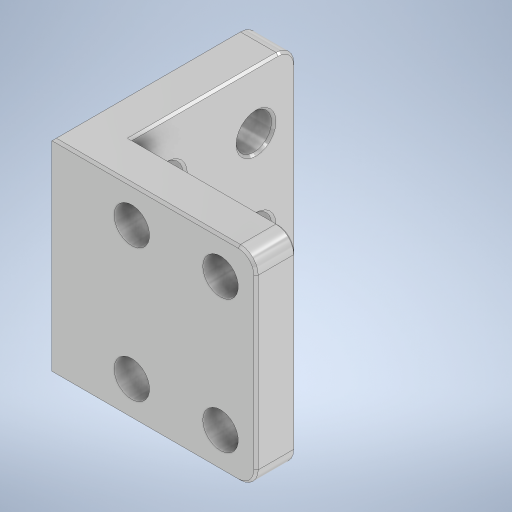
# Autodesk Inventor part: HUDSON-1-06 FRONT BUFFER BEAM ANGLE
Saved by Autodesk Inventor 2024.2 (Build 282272000, 272)
## iProperties
Created: 2024-10-05
Part Number: HUDSON-1-06 FRONT BUFFER BEAM ANGLE
Material: Generic
Document SubType Name: Modeling
Designer: Jimena Brenes
Density: 1 g/cm^3
Appearance: Aluminum - Dark
Author: Jimena Brenes
Autodesk Inventor part; units mm, degrees
ref_plane "YZ Plane" through (0, 0, 0) normal (1, 0, 0) x (0, 1, 0)
ref_plane "XZ Plane" through (0, 0, 0) normal (0, 1, 0) x (-1, 0, 0)
ref_plane "XY Plane" through (0, 0, 0) normal (0, 0, 1) x (1, 0, 0)
sketch "Sketch1" plane through (0, 0, 0) normal (0, 1, 0) x (-1, 0, 0)
  line L0 (0, 0) -> (0, -4.5)
  line L1 (0, 0) -> (23, 0)
  line L2 (23, 0) -> (23, -23)
  line L3 (23, -23) -> (18.5, -23)
  line L4 (0, -4.5) -> (18.5, -4.5)
  line L5 (18.5, -4.5) -> (18.5, -23)
  dimension "d0" = 4.5
  dimension "d1" = 23
  dimension "d2" = 23
  dimension "d3" = 4.5
  constraints: 12 end point, 3 perpendicular, 2 horizontal, 1 vertical
  measures "d0" distance of L0.start L0.end
  measures "d1" distance of L0.start L1.end
  measures "d2" distance of L1.end L2.end
  measures "d3" distance of L2.end L3.end
extrude "Extrusion1" add sketch "Sketch1" along normal blind 23
fillet "Fillet1" radius 2 4 edges at (-20.75, 23, -23) (-20.75, 0, -23) (0, 0, -2.25) (0, 23, -2.25)
sketch "Sketch2" plane through (-18.5, 0, -4.5) normal (0, 0, -1) x (-1, 0, 0)
  circle A0 centre (-14.5, 19) radius 2
  circle A1 centre (-4.5, 19) radius 2
  circle A2 centre (-4.5, 4) radius 2
  circle A3 centre (-14.5, 4) radius 2
  line L0 (-16.5, 23) -> (0, 23) projected
  line L1 (-16.5, 0) -> (0, 0) projected
  line L2 (-18.5, 2) -> (-18.5, 21) projected
  line L3 (4.5, 2) -> (4.5, 21) projected
  point P0 (-18.5, 0)
  dimension "d7" = 4
  dimension "d8" = 4
  dimension "d9" = 4
  dimension "d10" = 4
  dimension "d11" = 4
  dimension "d12" = 15
  dimension "d13" = 4
  dimension "d14" = 4
  dimension "d15" = 10
  dimension "d16" = 4
  dimension "d17" = 4
  dimension "d18" = 9
  dimension "d19" = 9
  constraints: 4 centre point
  measures "d7" diameter of A0
  measures "d8" diameter of A1
  measures "d9" diameter of A2
  measures "d10" diameter of A3
  measures "d11" distance from line of L0 A0.centre
  measures "d12" distance of A3.centre A0.centre
  measures "d13" distance from line of L1 A3.centre
  measures "d14" distance from line of L2 A3.centre
  measures "d15" distance of A3.centre A2.centre
  measures "d16" distance from line of L1 A2.centre
  measures "d17" distance from line of L0 A1.centre
  measures "d18" distance from line of L3 A1.centre
  measures "d19" distance from line of L3 A2.centre
hole "Hole1" at (-4, 19, -4.5) at (-4, 4, -4.5) at (-14, 19, -4.5) at (-14, 4, -4.5) direction (0, 0, 1) diameter 4 depth 4.5 tip angle 118
sketch "Sketch3" plane through (-18.5, 0, -4.5) normal (1, 0, 0) x (0, 0, -1)
  line L0 (4, 16.5) -> (14, 16.5) construction
  line L1 (14, 16.5) -> (14, 6.5) construction
  line L2 (14, 6.5) -> (4, 6.5) construction
  line L3 (4, 6.5) -> (4, 16.5) construction
  circle A0 centre (4, 16.5) radius 2
  circle A1 centre (14, 16.5) radius 2
  circle A2 centre (14, 6.5) radius 2
  circle A3 centre (4, 6.5) radius 2
  line L4 (0, 23) -> (16.5, 23) projected
  line L5 (-4.5, 2) -> (-4.5, 21) projected
  line L6 (18.5, 2) -> (18.5, 21) projected
  point P0 (-4.5, 0)
  dimension "d27" = 4
  dimension "d28" = 4
  dimension "d29" = 4
  dimension "d30" = 4
  dimension "d31" = 6.5
  dimension "d32" = 10
  dimension "d33" = 10
  dimension "d34" = 8.5
  dimension "d35" = 4.5
  constraints: 8 end point, 4 centre point, 4 coincident, 2 parallel, 1 horizontal, 1 perpendicular
  measures "d27" diameter of A0
  measures "d28" diameter of A1
  measures "d29" diameter of A2
  measures "d30" diameter of A3
  measures "d31" distance from line of L4 L0.end
  measures "d32" distance of L0.end L1.end
  measures "d33" distance of L2.end L1.end
  measures "d34" distance from line of L5 L0.start
  measures "d35" distance from line of L6 L1.end
hole "Hole2" at (-18.5, 16.5, -8.5) at (-18.5, 16.5, -18.5) at (-18.5, 6.5, -8.5) at (-18.5, 6.5, -18.5) direction (-1, 0, 0) diameter 4 depth 4.5 tip angle 118
chamfer "Chamfer1" distance 0.25 angle 45 28 edges at (-10.25, 23, -4.5) (-0.5858, 22.4142, -4.5) (0, 11.5, -4.5) (-0.5858, 0.5858, -4.5) (-10.25, 0, -4.5) (-12.5, 23, 0) (-0.5858, 22.4142, 0) (0, 11.5, 0) (-0.5858, 0.5858, 0) (-12.5, 0, 0) (-18.5, 23, -12.75) (-18.5, 22.4142, -22.4142) (-18.5, 11.5, -23) (-18.5, 0.5858, -22.4142) (-18.5, 0, -12.75) (-23, 23, -10.5) (-23, 22.4142, -22.4142) (-23, 11.5, -23) (-23, 0.5858, -22.4142) (-23, 0, -10.5) (-18.5, 16.5, -6.5) (-18.5, 16.5, -16.5) (-18.5, 6.5, -6.5) (-18.5, 6.5, -16.5) (-14, 17, -4.5) (-4, 17, -4.5) (-14, 2, -4.5) (-4, 2, -4.5)
body "Solid1"
